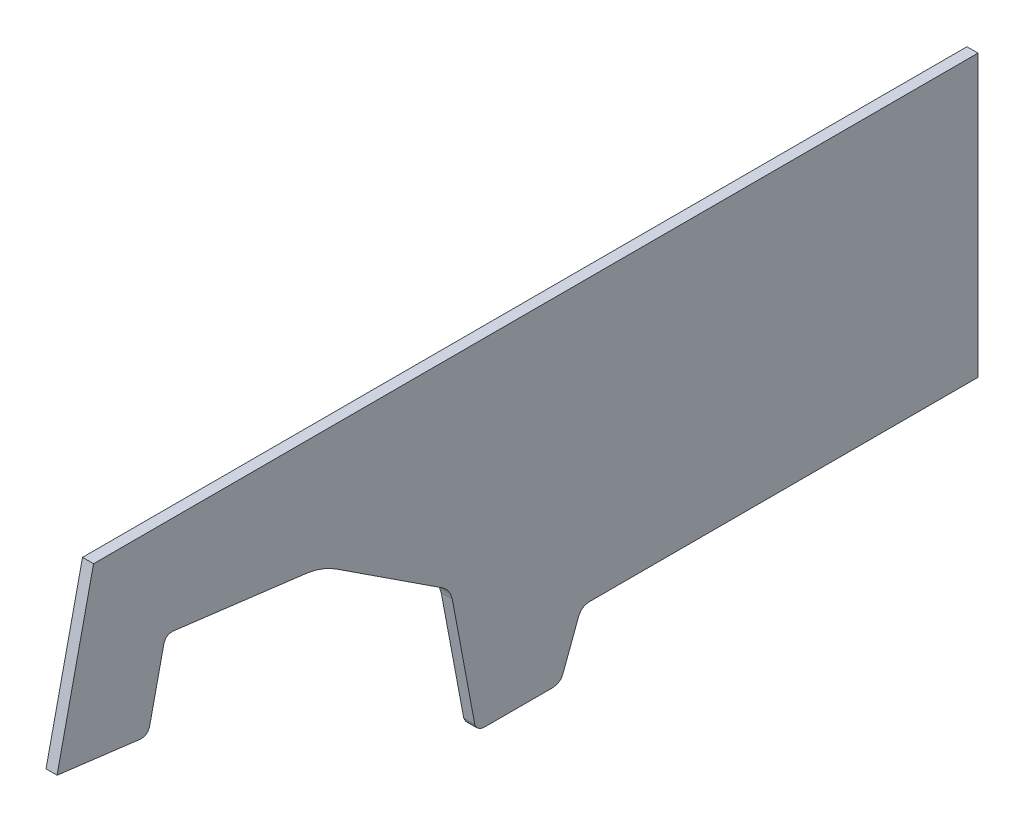
# Autodesk Inventor part: CUT PART A
Saved by Autodesk Inventor 2023.1 (Build 271208000, 208)
## iProperties
Created: 2022-11-02
Part Number: CUT PART A
Material: Generic
Document SubType Name: Modeling
Designer: GUT
Density: 1 g/cm^3
Appearance: Default
Author: GUT
Autodesk Inventor part; units mm, degrees
ref_plane "YZ Plane" through (0, 0, 0) normal (1, 0, 0) x (0, 1, 0)
ref_plane "XZ Plane" through (0, 0, 0) normal (0, 1, 0) x (-1, 0, 0)
ref_plane "XY Plane" through (0, 0, 0) normal (0, 0, 1) x (1, 0, 0)
sketch "Sketch1" plane through (0, 0, 0) normal (1, 0, 0) x (0, 1, 0)
  line L0 (609.6339, -895.1116) -> (609.6339, 705.0745)
  line L1 (101.6046, -895.1116) -> (609.6339, -895.1116)
  line L2 (101.6046, -191.1252) -> (101.6046, -895.1116)
  line L3 (12.7452, -144.2404) -> (89.1216, -172.8816)
  line L4 (0, -1.0766) -> (0, -127.1818)
  line L5 (609.6339, 705.0745) -> (311.1839, 771.1144)
  line L6 (311.1839, 771.1144) -> (292.2034, 619.2706)
  line L7 (303.0756, 603.8577) -> (421.3918, 577.677)
  arc A0 (292.2471, 619.62) -> (303.1676, 603.8374) centre (306.105, 617.5393) ccw
  line L8 (432.2642, 562.2641) -> (401.9995, 320.1465)
  line L9 (12.7343, 15.3075) -> (229.8814, 56.0932)
  line L10 (382.5827, 267.2032) -> (256.3621, 73.9914)
  arc A1 (432.2642, 562.2641) -> (421.3918, 577.677) centre (418.3657, 564.0012) ccw
  arc A2 (382.5827, 267.2032) -> (401.9995, 320.1465) centre (277.7698, 335.6752) ccw
  arc A3 (229.8814, 56.0932) -> (256.3621, 73.9914) centre (222.4584, 95.6141) ccw
  arc A4 (12.7343, 15.3075) -> (0, -1.0766) centre (16.907, -1.0766) ccw
  arc A5 (0, -127.1818) -> (12.7452, -144.2404) centre (17.7886, -127.1818) ccw
  arc A6 (101.6046, -191.1252) -> (89.1216, -172.8816) centre (82.366, -190.8966) ccw
  point P0 (0, 0)
  constraints: 22 end point, 14 point on circle, 7 centre point, 6 tangent, 2 point on line
extrude "Extrusion1" add sketch "Sketch1" along normal blind 20
body "Solid1"
